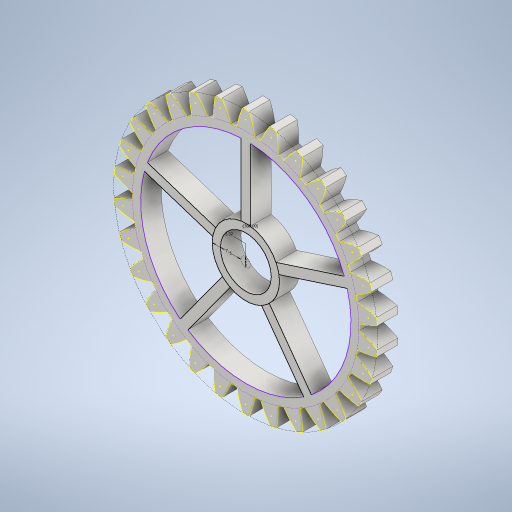
# Autodesk Inventor part: Spur Gear2
Saved by Autodesk Inventor 2023 (Build 270158000, 158)
## iProperties
CustomPartVersion: 0
Created: 2022-11-24
Part Number: Spur Gear2
Material: Steel
Document SubType Name: Modeling
Designer: shrey
Categories: <?xml version="1.0" encoding="UTF-16"?> <MemberInstance><Categories><FamilyTemplate><FamilyTemplateParameter ValueType="xs:double" Id="1" ObjectReferenceKey="da_z" ObjectType="kUserParameterObject"/><FamilyTemplateParameter ValueType="xs:double" Id="2" ObjectReferenceKey="da_b" ObjectType="kUserParameterObject"/><FamilyTemplateParameter ValueType="xs:double" Id="3" ObjectReferenceKey="da_beta" ObjectType="kUserParameterObject"/><FamilyTemplateParameter ValueType="xs:double" Id="4" ObjectReferenceKey="da_da" ObjectType="kUserParameterObject"/><FamilyTemplateParameter ValueType="xs:double" Id="5" ObjectReferenceKey="da_aw" ObjectType="kUserParameterObject"/><FamilyTemplateParameter ValueType="xs:string" Id="6" ObjectReferenceKey="EAIAABAAAACIAQAAAAAAAIAAAAAAAAAA" ObjectType="83910656" SubObjectId="SurfaceGeometry"/></FamilyTemplate><ParamToTemplateMap><ParamToTemplate CategoryParameter="//CategoryParameter[@InternalName='046C89C9-8512-4d59-83FE-43B91F4F132A']" TemplateParameter="1"/><ParamToTemplate CategoryParameter="//CategoryParameter[@InternalName='2552DF32-E462-4b46-AEBF-C6C7768E72AC']" TemplateParameter="2"/><ParamToTemplate CategoryParameter="//CategoryParameter[@InternalName='C9EE641D-15FC-4fae-A226-E94C4372FDD7']" TemplateParameter="3"/><ParamToTemplate><ParamToTemplate CategoryParameter="//CategoryParameter[@InternalName='00B6519A-459B-49c7-AD84-2E56D39A5744']" ConstantValue="0.000000"/></ParamToTemplate><ParamToTemplate><ParamToTemplate CategoryParameter="//CategoryParameter[@InternalName='04B31F0E-C7A6-4894-AA32-9629BEFACF47']" ConstantValue="1.000000"/></ParamToTemplate><ParamToTemplate><ParamToTemplate CategoryParameter="//CategoryParameter[@InternalName='43CBEC2E-7847-49e7-A936-2F7889FCB2D9']" ConstantValue="0.250000"/></ParamToTemplate><ParamToTemplate><ParamToTemplate CategoryParameter="//CategoryParameter[@InternalName='B1EFC894-105D-4ebd-86BF-FA20ED196853']" ConstantValue="0.350000"/></ParamToTemplate><ParamToTemplate><ParamToTemplate CategoryParameter="//CategoryParameter[@InternalName='51175063-3D10-4879-93E8-6246FE8B403D']" ConstantValue="2060000000.000000"/></ParamToTemplate><ParamToTemplate><ParamToTemplate CategoryParameter="//CategoryParameter[@InternalName='A3A52E27-4454-46a9-B0BD-C932399B70AF']" ConstantValue="0.300000"/></ParamToTemplate><ParamToTemplate><ParamToTemplate CategoryParameter="//CategoryParameter[@InternalName='91B76062-C214-41d9-B1B9-14D2AB99603D']" ConstantValue="0.200000"/></ParamToTemplate><ParamToTemplate><ParamToTemplate CategoryParameter="//CategoryParameter[@InternalName='374E806E-8B8A-4dda-A9AA-1039D6500AD2']" ConstantValue="5.000000"/></ParamToTemplate><ParamToTemplate><ParamToTemplate CategoryParameter="//CategoryParameter[@InternalName='2D373A89-B862-43d6-8D0B-0CBF12AB9F6C']" ConstantValue="0.349066"/></ParamToTemplate><ParamToTemplate CategoryParameter="//CategoryParameter[@InternalName='37777632-D6A2-4fac-9D53-DB8ACD95C989']" TemplateParameter="4"/><ParamToTemplate CategoryParameter="//CategoryParameter[@InternalName='FD1017F1-B727-4f7e-9707-0F86F1FF9423']" TemplateParameter="5"/><ParamToTemplate><ParamToTemplate CategoryParameter="//CategoryParameter[@InternalName='9E1B4470-B2D3-4ff1-B813-535BB4CDF51A']" ConstantValue="3520000.000000"/></ParamToTemplate><ParamToTemplate><ParamToTemplate CategoryParameter="//CategoryParameter[@InternalName='F8452263-BFF6-458c-9FB1-07C4B99E95CD']" ConstantValue="11400000.000000"/></ParamToTemplate><ParamToTemplate><ParamToTemplate CategoryParameter="//CategoryParameter[@InternalName='3E3BB259-FD49-497f-8171-6EBC954A3479']" ConstantValue="2.000000"/></ParamToTemplate><ParamToTemplate CategoryParameter="//CategoryParameter[@InternalName='27C3BAF2-7550-4e4b-AE2C-0DB134B7D9B7']" TemplateParameter="6"/></ParamToTemplateMap><Category DisplayName="Gear" InternalName="DC85795E-93AB-48d5-8EEE-5A27447B64BD" Mnemonic="Gear"><CategoryParameter DisplayName="z" InternalName="046C89C9-8512-4d59-83FE-43B91F4F132A" Mnemonic="z"/><CategoryParameter DisplayName="b" InternalName="2552DF32-E462-4b46-AEBF-C6C7768E72AC" Mnemonic="b"/><CategoryParameter DisplayName="||b|" InternalName="C9EE641D-15FC-4fae-A226-E94C4372FDD7" Mnemonic="beta"/><CategoryParameter DisplayName="x" InternalName="00B6519A-459B-49c7-AD84-2E56D39A5744" Mnemonic="x"/><CategoryParameter DisplayName="a*" InternalName="04B31F0E-C7A6-4894-AA32-9629BEFACF47" Mnemonic="a"/><CategoryParameter DisplayName="c*" InternalName="43CBEC2E-7847-49e7-A936-2F7889FCB2D9" Mnemonic="c"/><CategoryParameter DisplayName="r|.f|*" InternalName="B1EFC894-105D-4ebd-86BF-FA20ED196853" Mnemonic="rf"/><CategoryParameter DisplayName="E" InternalName="51175063-3D10-4879-93E8-6246FE8B403D" Mnemonic="E"/><CategoryParameter DisplayName="||m|" InternalName="A3A52E27-4454-46a9-B0BD-C932399B70AF" Mnemonic="mi"/><Category DisplayName="SpurGear" InternalName="26C5A22E-A91E-4dfd-A3B3-23CCAFAE1764" Mnemonic="SpurGear"><CategoryParameter DisplayName="m" InternalName="91B76062-C214-41d9-B1B9-14D2AB99603D" Mnemonic="m"/><CategoryParameter DisplayName="P" InternalName="374E806E-8B8A-4dda-A9AA-1039D6500AD2" Mnemonic="PP"/><CategoryParameter DisplayName="||a|" InternalName="2D373A89-B862-43d6-8D0B-0CBF12AB9F6C" Mnemonic="alpha"/><CategoryParameter DisplayName="d|.a|" InternalName="37777632-D6A2-4fac-9D53-DB8ACD95C989" Mnemonic="da"/><CategoryParameter DisplayName="a|.w|" InternalName="FD1017F1-B727-4f7e-9707-0F86F1FF9423" Mnemonic="aw"/><CategoryParameter DisplayName="||s||.Flim|" InternalName="9E1B4470-B2D3-4ff1-B813-535BB4CDF51A" Mnemonic="sFlim"/><CategoryParameter DisplayName="||s||.Hlim|" InternalName="F8452263-BFF6-458c-9FB1-07C4B99E95CD" Mnemonic="sHlim"/><CategoryParameter DisplayName="type" InternalName="3E3BB259-FD49-497f-8171-6EBC954A3479" Mnemonic="type"/><CategoryParameter DisplayName="PitchDiameter" InternalName="27C3BAF2-7550-4e4b-AE2C-0DB134B7D9B7" Mnemonic="IDS_PITCHDIAM"/></Category></Category></Categories></MemberInstance>
Density: 1 g/cm^3
Appearance: Steel
Author: shrey
Autodesk Inventor part; units mm, degrees
sketch "Sketch1" plane through (0, 0, 0) normal (0, 0, 1) x (1, 0, 0)
  circle A0 centre (0, 0) radius 32
  dimension "d0" = 64
  constraints: 1 centre point
  measures "d0" diameter of A0
extrude "Extrusion1" add sketch "Sketch1" along normal blind 5
ref_plane "Work Plane2" through (0, 0, 2.5) normal (0, 0, 1) x (1, 0, 0)
sketch "Sketch2" plane through (0, 0, 0) normal (0, 0, -1) x (-1, 0, 0)
  circle A0 centre (0, 0) radius 32 projected
  circle A1 centre (0, 0) radius 30
  dimension "d3" = 60
  constraints: 1 centre point, 1 coincident
  measures "d3" diameter of A1
surface extrude "Pitch Diameter" sketch "Sketch2" against normal through all shown no curves A1
ref_plane "Work Plane8" through (0, 0, 0) normal (0.9945219, 0.1045285, 0) x (0, 0, 1)
ref_plane "Work Plane9" through (0, 0, 0) normal (1, 0, 0) x (0, 1, 0)
spur gear teeth "Spur Gear" teeth 30 pitch diameter 60 tip diameter 64 root diameter 55 face width 5 start plane through (0, 0, 0) normal (0, 0, -1) x (-1, 0, 0)
sketch "Sketch3" plane through (0, 0, 5) normal (0, 0, 1) x (1, 0, 0)
  arc A0 (-7.4703, 31.1158) -> (-7.8104, 26.3675) centre (12.177, 27.322) ccw projected
  arc A1 (-7.8104, 26.3675) -> (-9.1797, 25.9226) centre (0, 0) ccw projected
  arc A2 (-9.1797, 25.9226) -> (-12.2459, 29.5641) centre (-25.9108, 14.9465) ccw projected
  arc A3 (-12.2459, 29.5641) -> (-13.7764, 28.8827) centre (0, 0) ccw projected
  arc A4 (-13.7764, 28.8827) -> (-13.1219, 24.1675) centre (6.2303, 29.2567) ccw projected
  arc A5 (-13.1219, 24.1675) -> (-14.3687, 23.4476) centre (0, 0) ccw projected
  arc A6 (-14.3687, 23.4476) -> (-18.125, 26.372) centre (-28.4522, 9.2327) ccw projected
  arc A7 (-18.125, 26.372) -> (-19.4804, 25.3873) centre (0, 0) ccw projected
  arc A8 (-19.4804, 25.3873) -> (-17.8598, 20.9112) centre (0.0114, 29.9127) ccw projected
  arc A9 (-17.8598, 20.9112) -> (-18.9298, 19.9478) centre (0, 0) ccw projected
  arc A10 (-18.9298, 19.9478) -> (-23.212, 22.0273) centre (-29.75, 3.1154) ccw projected
  arc A11 (-23.212, 22.0273) -> (-24.333, 20.7823) centre (0, 0) ccw projected
  arc A12 (-24.333, 20.7823) -> (-21.8172, 16.7409) centre (-6.2081, 29.2614) ccw projected
  arc A13 (-21.8172, 16.7409) -> (-22.6635, 15.5762) centre (0, 0) ccw projected
  arc A14 (-22.6635, 15.5762) -> (-27.2845, 16.72) centre (-29.7476, -3.138) ccw projected
  arc A15 (-27.2845, 16.72) -> (-28.1221, 15.2691) centre (0, 0) ccw projected
  arc A16 (-28.1221, 15.2691) -> (-24.8211, 11.8391) centre (-12.1562, 27.3312) ccw projected
  arc A17 (-24.8211, 11.8391) -> (-25.4067, 10.5238) centre (0, 0) ccw projected
  arc A18 (-25.4067, 10.5238) -> (-30.1645, 10.6818) centre (-28.4451, -9.2543) ccw projected
  arc A19 (-30.1645, 10.6818) -> (-30.6822, 9.0885) centre (0, 0) ccw projected
  arc A20 (-30.6822, 9.0885) -> (-26.7402, 6.4197) centre (-17.573, 24.2065) ccw projected
  arc A21 (-26.7402, 6.4197) -> (-27.0395, 5.0115) centre (0, 0) ccw projected
  arc A22 (-27.0395, 5.0115) -> (-31.7262, 4.1768) centre (-25.8995, -14.9662) ccw projected
  arc A23 (-31.7262, 4.1768) -> (-31.9014, 2.5107) centre (0, 0) ccw projected
  arc A24 (-31.9014, 2.5107) -> (-27.4906, 0.7199) centre (-22.2218, 20.0239) ccw projected
  arc A25 (-27.4906, 0.7199) -> (-27.4906, -0.7199) centre (0, 0) ccw projected
  arc A26 (-27.4906, -0.7199) -> (-31.9014, -2.5107) centre (-22.2218, -20.0239) ccw projected
  arc A27 (-31.9014, -2.5107) -> (-31.7262, -4.1768) centre (0, 0) ccw projected
  arc A28 (-31.7262, -4.1768) -> (-27.0395, -5.0115) centre (-25.8995, 14.9662) ccw projected
  arc A29 (-27.0395, -5.0115) -> (-26.7402, -6.4197) centre (0, 0) ccw projected
  arc A30 (-26.7402, -6.4197) -> (-30.6822, -9.0885) centre (-17.573, -24.2065) ccw projected
  arc A31 (-30.6822, -9.0885) -> (-30.1645, -10.6818) centre (0, 0) ccw projected
  arc A32 (-30.1645, -10.6818) -> (-25.4067, -10.5238) centre (-28.4451, 9.2543) ccw projected
  arc A33 (-25.4067, -10.5238) -> (-24.8211, -11.8391) centre (0, 0) ccw projected
  arc A34 (-24.8211, -11.8391) -> (-28.1221, -15.2691) centre (-12.1562, -27.3312) ccw projected
  arc A35 (-28.1221, -15.2691) -> (-27.2845, -16.72) centre (0, 0) ccw projected
  arc A36 (-27.2845, -16.72) -> (-22.6635, -15.5762) centre (-29.7476, 3.138) ccw projected
  arc A37 (-22.6635, -15.5762) -> (-21.8172, -16.7409) centre (0, 0) ccw projected
  arc A38 (-21.8172, -16.7409) -> (-24.333, -20.7823) centre (-6.2081, -29.2614) ccw projected
  arc A39 (-24.333, -20.7823) -> (-23.212, -22.0273) centre (0, 0) ccw projected
  arc A40 (-23.212, -22.0273) -> (-18.9298, -19.9478) centre (-29.75, -3.1154) ccw projected
  arc A41 (-18.9298, -19.9478) -> (-17.8598, -20.9112) centre (0, 0) ccw projected
  arc A42 (-17.8598, -20.9112) -> (-19.4804, -25.3873) centre (0.0114, -29.9127) ccw projected
  arc A43 (-19.4804, -25.3873) -> (-18.125, -26.372) centre (0, 0) ccw projected
  arc A44 (-18.125, -26.372) -> (-14.3687, -23.4476) centre (-28.4522, -9.2327) ccw projected
  arc A45 (-14.3687, -23.4476) -> (-13.1219, -24.1675) centre (0, 0) ccw projected
  arc A46 (-13.1219, -24.1675) -> (-13.7764, -28.8827) centre (6.2303, -29.2567) ccw projected
  arc A47 (-13.7764, -28.8827) -> (-12.2459, -29.5641) centre (0, 0) ccw projected
  arc A48 (-12.2459, -29.5641) -> (-9.1797, -25.9226) centre (-25.9108, -14.9465) ccw projected
  arc A49 (-9.1797, -25.9226) -> (-7.8104, -26.3675) centre (0, 0) ccw projected
  arc A50 (-7.8104, -26.3675) -> (-7.4703, -31.1158) centre (12.177, -27.322) ccw projected
  arc A51 (-7.4703, -31.1158) -> (-5.8315, -31.4642) centre (0, 0) ccw projected
  arc A52 (-5.8315, -31.4642) -> (-3.5895, -27.2647) centre (-22.2371, -20.007) ccw projected
  arc A53 (-3.5895, -27.2647) -> (-2.1576, -27.4152) centre (0, 0) ccw projected
  arc A54 (-2.1576, -27.4152) -> (-0.8377, -31.989) centre (17.5914, -24.1932) ccw projected
  arc A55 (-0.8377, -31.989) -> (0.8377, -31.989) centre (0, 0) ccw projected
  arc A56 (0.8377, -31.989) -> (2.1576, -27.4152) centre (-17.5914, -24.1932) ccw projected
  arc A57 (2.1576, -27.4152) -> (3.5895, -27.2647) centre (0, 0) ccw projected
  arc A58 (3.5895, -27.2647) -> (5.8315, -31.4642) centre (22.2371, -20.007) ccw projected
  arc A59 (5.8315, -31.4642) -> (7.4703, -31.1158) centre (0, 0) ccw projected
  arc A60 (7.4703, -31.1158) -> (7.8104, -26.3675) centre (-12.177, -27.322) ccw projected
  arc A61 (7.8104, -26.3675) -> (9.1797, -25.9226) centre (0, 0) ccw projected
  arc A62 (9.1797, -25.9226) -> (12.2459, -29.5641) centre (25.9108, -14.9465) ccw projected
  arc A63 (12.2459, -29.5641) -> (13.7764, -28.8827) centre (0, 0) ccw projected
  arc A64 (13.7764, -28.8827) -> (13.1219, -24.1675) centre (-6.2303, -29.2567) ccw projected
  arc A65 (13.1219, -24.1675) -> (14.3687, -23.4476) centre (0, 0) ccw projected
  arc A66 (14.3687, -23.4476) -> (18.125, -26.372) centre (28.4522, -9.2327) ccw projected
  arc A67 (18.125, -26.372) -> (19.4804, -25.3873) centre (0, 0) ccw projected
  arc A68 (19.4804, -25.3873) -> (17.8598, -20.9112) centre (-0.0114, -29.9127) ccw projected
  arc A69 (17.8598, -20.9112) -> (18.9298, -19.9478) centre (0, 0) ccw projected
  arc A70 (18.9298, -19.9478) -> (23.212, -22.0273) centre (29.75, -3.1154) ccw projected
  arc A71 (23.212, -22.0273) -> (24.333, -20.7823) centre (0, 0) ccw projected
  arc A72 (24.333, -20.7823) -> (21.8172, -16.7409) centre (6.2081, -29.2614) ccw projected
  arc A73 (21.8172, -16.7409) -> (22.6635, -15.5762) centre (0, 0) ccw projected
  arc A74 (22.6635, -15.5762) -> (27.2845, -16.72) centre (29.7476, 3.138) ccw projected
  arc A75 (27.2845, -16.72) -> (28.1221, -15.2691) centre (0, 0) ccw projected
  arc A76 (28.1221, -15.2691) -> (24.8211, -11.8391) centre (12.1562, -27.3312) ccw projected
  arc A77 (24.8211, -11.8391) -> (25.4067, -10.5238) centre (0, 0) ccw projected
  arc A78 (25.4067, -10.5238) -> (30.1645, -10.6818) centre (28.4451, 9.2543) ccw projected
  arc A79 (30.1645, -10.6818) -> (30.6822, -9.0885) centre (0, 0) ccw projected
  arc A80 (30.6822, -9.0885) -> (26.7402, -6.4197) centre (17.573, -24.2065) ccw projected
  arc A81 (26.7402, -6.4197) -> (27.0395, -5.0115) centre (0, 0) ccw projected
  arc A82 (27.0395, -5.0115) -> (31.7262, -4.1768) centre (25.8995, 14.9662) ccw projected
  arc A83 (31.7262, -4.1768) -> (31.9014, -2.5107) centre (0, 0) ccw projected
  arc A84 (31.9014, -2.5107) -> (27.4906, -0.7199) centre (22.2218, -20.0239) ccw projected
  arc A85 (27.4906, -0.7199) -> (27.4906, 0.7199) centre (0, 0) ccw projected
  arc A86 (27.4906, 0.7199) -> (31.9014, 2.5107) centre (22.2218, 20.0239) ccw projected
  arc A87 (31.9014, 2.5107) -> (31.7262, 4.1768) centre (0, 0) ccw projected
  arc A88 (31.7262, 4.1768) -> (27.0395, 5.0115) centre (25.8995, -14.9662) ccw projected
  arc A89 (27.0395, 5.0115) -> (26.7402, 6.4197) centre (0, 0) ccw projected
  arc A90 (26.7402, 6.4197) -> (30.6822, 9.0885) centre (17.573, 24.2065) ccw projected
  arc A91 (30.6822, 9.0885) -> (30.1645, 10.6818) centre (0, 0) ccw projected
  arc A92 (30.1645, 10.6818) -> (25.4067, 10.5238) centre (28.4451, -9.2543) ccw projected
  arc A93 (25.4067, 10.5238) -> (24.8211, 11.8391) centre (0, 0) ccw projected
  arc A94 (24.8211, 11.8391) -> (28.1221, 15.2691) centre (12.1562, 27.3312) ccw projected
  arc A95 (28.1221, 15.2691) -> (27.2845, 16.72) centre (0, 0) ccw projected
  arc A96 (27.2845, 16.72) -> (22.6635, 15.5762) centre (29.7476, -3.138) ccw projected
  arc A97 (22.6635, 15.5762) -> (21.8172, 16.7409) centre (0, 0) ccw projected
  arc A98 (21.8172, 16.7409) -> (24.333, 20.7823) centre (6.2081, 29.2614) ccw projected
  arc A99 (24.333, 20.7823) -> (23.212, 22.0273) centre (0, 0) ccw projected
  arc A100 (23.212, 22.0273) -> (18.9298, 19.9478) centre (29.75, 3.1154) ccw projected
  arc A101 (18.9298, 19.9478) -> (17.8598, 20.9112) centre (0, 0) ccw projected
  arc A102 (17.8598, 20.9112) -> (19.4804, 25.3873) centre (-0.0114, 29.9127) ccw projected
  arc A103 (19.4804, 25.3873) -> (18.125, 26.372) centre (0, 0) ccw projected
  arc A104 (18.125, 26.372) -> (14.3687, 23.4476) centre (28.4522, 9.2327) ccw projected
  arc A105 (14.3687, 23.4476) -> (13.1219, 24.1675) centre (0, 0) ccw projected
  arc A106 (13.1219, 24.1675) -> (13.7764, 28.8827) centre (-6.2303, 29.2567) ccw projected
  arc A107 (13.7764, 28.8827) -> (12.2459, 29.5641) centre (0, 0) ccw projected
  arc A108 (12.2459, 29.5641) -> (9.1797, 25.9226) centre (25.9108, 14.9465) ccw projected
  arc A109 (9.1797, 25.9226) -> (7.8104, 26.3675) centre (0, 0) ccw projected
  arc A110 (7.8104, 26.3675) -> (7.4703, 31.1158) centre (-12.177, 27.322) ccw projected
  arc A111 (7.4703, 31.1158) -> (5.8315, 31.4642) centre (0, 0) ccw projected
  arc A112 (5.8315, 31.4642) -> (3.5895, 27.2647) centre (22.2371, 20.007) ccw projected
  arc A113 (3.5895, 27.2647) -> (2.1576, 27.4152) centre (0, 0) ccw projected
  arc A114 (2.1576, 27.4152) -> (0.8377, 31.989) centre (-17.5914, 24.1932) ccw projected
  arc A115 (0.8377, 31.989) -> (-0.8377, 31.989) centre (0, 0) ccw projected
  arc A116 (-0.8377, 31.989) -> (-2.1576, 27.4152) centre (17.5914, 24.1932) ccw projected
  arc A117 (-2.1576, 27.4152) -> (-3.5895, 27.2647) centre (0, 0) ccw projected
  arc A118 (-3.5895, 27.2647) -> (-5.8315, 31.4642) centre (-22.2371, 20.007) ccw projected
  arc A119 (-5.8315, 31.4642) -> (-7.4703, 31.1158) centre (0, 0) ccw projected
  circle A120 centre (0, 0) radius 32 construction
  arc A121 (3.5895, 27.2647) -> (2.1576, 27.4152) centre (0, 0) ccw construction
  circle A122 centre (0, 0) radius 27.5 construction
  circle A123 centre (0, 0) radius 1.16 construction
  circle A124 centre (0, 0) radius 8.16
  line L0 (-1.16, 8.0771) -> (-1.16, 25.4736)
  line L1 (1.16, 8.0771) -> (1.16, 25.4736)
  line L2 (-7.3233, 3.5992) -> (-23.8684, 8.975)
  line L3 (-8.0403, 1.3927) -> (-24.5853, 6.7686)
  line L4 (-5.6861, -5.8527) -> (-15.9115, -19.9267)
  line L5 (-3.8092, -7.2164) -> (-14.0345, -21.2904)
  line L6 (3.8092, -7.2164) -> (14.0345, -21.2904)
  line L7 (5.6861, -5.8527) -> (15.9115, -19.9267)
  line L8 (8.0403, 1.3927) -> (24.5853, 6.7686)
  line L9 (7.3233, 3.5992) -> (23.8684, 8.975)
  arc A125 (23.8684, 8.975) -> (1.16, 25.4736) centre (0, 0) ccw
  arc A126 (15.9115, -19.9267) -> (24.5853, 6.7686) centre (0, 0) ccw
  arc A127 (-14.0345, -21.2904) -> (14.0345, -21.2904) centre (0, 0) ccw
  arc A128 (-1.16, 25.4736) -> (-23.8684, 8.975) centre (0, 0) ccw
  arc A129 (-24.5853, 6.7686) -> (-15.9115, -19.9267) centre (0, 0) ccw
  circle A130 centre (0, 0) radius 6.16
  point P0 (8.0403, 1.3927)
  point P1 (5.6861, -5.8527)
  point P2 (3.8092, -7.2164)
  point P3 (-3.8092, -7.2164)
  point P4 (-8.0403, 1.3927)
  point P5 (-7.3233, 3.5992)
  point P6 (7.3233, 3.5992)
  dimension "d49" = 2.32
  dimension "d50" = 7
  dimension "d54" = 360
  dimension "d58" = 5
  constraints: 20 end point, 12 point on circle, 10 centre point, 3 coincident, 2 tangent, 2 vertical, 1 concentric, 31 other
  measures "d49" diameter of A123
  measures "d50" radial gap between concentric circles of A123 A124
  measures "d58" radial gap between concentric circles of A123 A130
extrude "Extrusion2" cut sketch "Sketch3" against normal through all contours A124 L8 A126 L7 | A124 L1 A125 L9 | L6 A127 L5 A124 | A124 L2 A128 L0 | L4 A129 L3 A124 | A130
equation "\"d0\" = da_da"
equation "\"d3\" = da_d"
equation "\"da_da\" = 64"
equation "\"da_d\" = 60"
body "Solid1"
body "Srf1"
